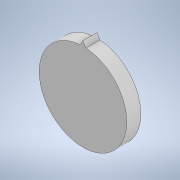
# Autodesk Inventor part: 18_ref
Saved by Autodesk Inventor 2021 (Build 250183000, 183)
## iProperties
Created: 2021-03-25
Part Number: 18_ref
Material: Generic
Document SubType Name: Modeling
Designer: lucia
Density: 1 g/cm^3
Appearance: Default
Author: lucia
Autodesk Inventor part; units mm, degrees
ref_plane "YZ Plane" through (0, 0, 0) normal (1, 0, 0) x (0, 1, 0)
ref_plane "XZ Plane" through (0, 0, 0) normal (0, 1, 0) x (-1, 0, 0)
ref_plane "XY Plane" through (0, 0, 0) normal (0, 0, 1) x (1, 0, 0)
sketch "Sketch1" plane through (0, 0, 0) normal (0, 0, 1) x (1, 0, 0)
  circle A0 centre (0, 0) radius 39.624
  line L0 (-2.54, 39.5425) -> (0, 43.9419)
  line L1 (0, 43.9419) -> (2.54, 39.5425)
  line L2 (2.54, 39.5425) -> (-2.54, 39.5425)
  dimension "d0" = 79.248
  dimension "d3" = 5.08
  constraints: 6 end point, 2 equal length, 2 point on circle, 1 centre point, 1 coincident, 1 horizontal
  measures "d0" diameter of A0
  measures "d3" distance of L1.end L0.start
extrude "Extrusion1" add sketch "Sketch1" against normal blind 12.7
equation "\"d0\" = 19.812 * scale"
equation "\"d3\" = 1.27 * scale"
equation "\"d1\" = 3.175 * scale"
equation "\"scale\" = 4"
body "Solid1"
